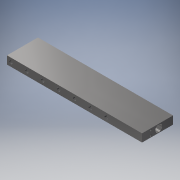
# Autodesk Inventor part: Ventilblock_4_links
Saved by Autodesk Inventor 2018 (Build 220112000, 112)
## iProperties
Created: 2011-11-24
Part Number: Ventilblock_4_links
Document SubType Name: Modeling
Designer: Neef
Density: 8 g/cm^3
Material: Stainless Steel
Appearance: Semi-Polished
Author: Neef
Autodesk Inventor part; units mm, degrees
ref_plane "YZ Plane" through (0, 0, 0) normal (1, 0, 0) x (0, 1, 0)
ref_plane "XZ Plane" through (0, 0, 0) normal (0, 1, 0) x (-1, 0, 0)
ref_plane "XY Plane" through (0, 0, 0) normal (0, 0, 1) x (1, 0, 0)
sketch "Skizze1" plane through (0, 0, 0) normal (0, 0, 1) x (1, 0, 0)
  line L0 (-85, 19.5) -> (85, 19.5)
  line L1 (85, 19.5) -> (85, -19.5)
  line L2 (85, -19.5) -> (-85, -19.5)
  line L3 (-85, -19.5) -> (-85, 19.5)
  line L4 (0, 27.3) -> (0, -27.3) projected
  line L5 (-119, 0) -> (119, 0) projected
  point P0 (0, 19.5)
  point P1 (85, 0)
  dimension "d0" = 39
  dimension "d1" = 170
  constraints: 8 end point, 2 midpoint, 2 parallel, 2 point on line, 1 horizontal, 1 perpendicular
  measures "d0" distance of L0.end L1.end
  measures "d1" distance of L0.start L0.end
extrude "Extrusion1" add sketch "Skizze1" along normal blind 10
sketch "Skizze6" plane through (0, 0, 0) normal (0, 0, -1) x (-1, 0, 0)
  line L0 (-85, -19.5) -> (85, -19.5) projected
  line L1 (85, -19.5) -> (85, 19.5) projected
  point P0 (80, -5.7)
  point P1 (80, -0.7)
  dimension "d77" = 5
  dimension "d78" = 5
  dimension "d79" = 18.8
  dimension "d80" = 13.8
  measures "d77" distance from line of L1 point (80, -5.7)
  measures "d78" distance from line of L1 point (80, -0.7)
  measures "d79" distance from line of L0 point (80, -0.7)
  measures "d80" distance from line of L0 point (80, -5.7)
hole "Bohrung7" at (-80, -5.7, 0) at (-80, -0.7, 0) direction (0, 0, 1) diameter 1.2 depth 5 tip angle 118
sketch "Skizze7" plane through (0, 0, 0) normal (0, 0, -1) x (-1, 0, 0)
  circle A0 centre (80, -5.7) radius 0.6 projected
  line L0 (-85, -19.5) -> (85, -19.5) projected
  point P0 (76.75, -4)
  point P1 (83.25, -4)
  dimension "d88" = 15.5
  dimension "d89" = 15.5
  dimension "d90" = 3.25
  dimension "d91" = 3.25
  measures "d88" distance from line of L0 point (83.25, -4)
  measures "d89" distance from line of L0 point (76.75, -4)
  measures "d90" horizontal distance of A0.centre point (83.25, -4)
  measures "d91" horizontal distance of A0.centre point (76.75, -4)
hole "Bohrung8" at (-76.75, -4, 0) at (-83.25, -4, 0) direction (0, 0, 1) diameter 1.221 depth 7 tip angle 118 thread size "M1.6x0.35" class "6H" standard "ISO Metric profile"
hole "Bohrung9" at (-80, -19.5, 5) direction (0, 1, 0) diameter 2 depth 14 tip angle 118
hole "Bohrung10" at (-80, -19.5, 5) direction (0, 1, 0) diameter 4.134 depth 7 tip angle 118 thread size "M5x0.8" class "6H" standard "ISO Metric profile"
pattern_linear "Rechteckige Anordnung3" count 7 spacing 20 along (1, 0, 0) of "Bohrung10", "Bohrung9", "Bohrung8", "Bohrung7"
sketch "Skizze11" plane through (-85, -19.5, 0) normal (-1, 0, 0) x (0, 0, 1)
  line L0 (10, 0) -> (10, 39) projected
  line L1 (0, 0) -> (0, 39) projected
  line L2 (0, 39) -> (10, 39) projected
  point P0 (0, 19.5)
  point P1 (8, 11)
  point P2 (2, 11)
  dimension "d255" = 2
  dimension "d256" = 2
  dimension "d264" = 28
  dimension "d265" = 28
  measures "d255" distance from line of L1 point (2, 11)
  measures "d256" distance from line of L0 point (8, 11)
  measures "d264" distance from line of L2 point (8, 11)
  measures "d265" distance from line of L2 point (2, 11)
hole "Bohrung25" at (-85, -8.5, 8) at (-85, -8.5, 2) direction (1, 0, 0) diameter 2.459 depth 12 tip angle 118 thread size "M3x0.5" class "6H" standard "ISO Metric profile"
sketch "Skizze12" plane through (85, -19.5, 0) normal (1, 0, 0) x (0, 0, -1)
  circle A0 centre (-2, 11) radius 1.2295 projected
  circle A1 centre (-8, 11) radius 1.2295 projected
  point P0 (0, 19.5)
  constraints: 2 coincident
hole "Bohrung26" at (85, -8.5, 8) at (85, -8.5, 2) direction (-1, 0, 0) diameter 2.459 depth 12 tip angle 118 thread size "M3x0.5" class "6H" standard "ISO Metric profile"
sketch "Skizze14" plane through (85, -19.5, 0) normal (1, 0, 0) x (0, 0, -1)
  line L0 (0, 39) -> (0, 0) projected
  line L1 (0, 39) -> (-10, 39) projected
  circle A0 centre (-5, 21) radius 4 construction
  line L2 (-7, 16.1105) -> (0, 16.1105) construction
  line L3 (-7, 14.8895) -> (0, 14.8895) construction
  point P0 (0, 19.5)
  dimension "d274" = 8
  dimension "d276" = 5
  dimension "d278" = 18
  constraints: 1 centre point, 1 coincident
  measures "d274" diameter of A0
  measures "d276" distance from line of L0 point (-5, 21)
  measures "d278" distance from line of point (-5, 21) L1
hole "Bohrung27" at (85, 1.5, 5) direction (-1, 0, 0) diameter 8 depth 166 tip angle 135
hole "Bohrung28" at (85, 1.5, 5) direction (-1, 0, 0) diameter 8.6 depth 12 tip angle 135
equation "\"d89\" = d88"
equation "\"d91\" = d90"
equation "\"d256\" = d255"
equation "\"d265\" = d264"
